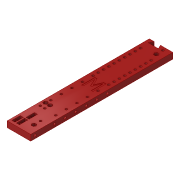
# Autodesk Inventor part: Coupler extension arm motor
Saved by Autodesk Inventor 2020 (Build 240168000, 168)
## iProperties
Created: 2019-10-02
Part Number: Coupler extension arm motor
Material: Generic
Document SubType Name: Modeling
Designer: ball
Density: 1 g/cm^3
Appearance: Default
Author: ball
Autodesk Inventor part; units mm, degrees
ref_plane "YZ Plane" through (0, 0, 0) normal (1, 0, 0) x (0, 1, 0)
ref_plane "XZ Plane" through (0, 0, 0) normal (0, 1, 0) x (-1, 0, 0)
ref_plane "XY Plane" through (0, 0, 0) normal (0, 0, 1) x (1, 0, 0)
sketch "Sketch1" plane through (0, 0, 0) normal (0, 1, 0) x (-1, 0, 0)
  line L0 (0, 0) -> (35.5, 0)
  line L1 (35.5, 0) -> (35.5, -215)
  line L2 (35.5, -215) -> (0, -215)
  line L3 (0, -215) -> (0, 0)
  dimension "d0" = 35.5
  dimension "d1" = 215
  constraints: 8 end point, 2 parallel, 1 horizontal, 1 perpendicular
  measures "d0" distance of L1.end L2.end
  measures "d1" distance of L0.end L1.end
extrude "BlockShape" add sketch "Sketch1" along normal blind 9
sketch "Sketch2" plane through (0, 9, 0) normal (0, 1, 0) x (1, 0, 0)
  circle A0 centre (-10, 15) radius 3.25 construction
  line L0 (-35.5, 0) -> (0, 0) projected
  line L1 (0, 0) -> (0, 215) projected
  line L2 (-13.25, 15) -> (-11.625, 17.8146)
  line L3 (-11.625, 17.8146) -> (-8.375, 17.8146)
  line L4 (-8.375, 17.8146) -> (-6.75, 15)
  line L5 (-6.75, 15) -> (-8.375, 12.1854)
  line L6 (-8.375, 12.1854) -> (-11.625, 12.1854)
  line L7 (-11.625, 12.1854) -> (-13.25, 15)
  circle A1 centre (-10, 200) radius 3.25 construction
  line L8 (-13.25, 200) -> (-11.625, 202.8146)
  line L9 (-11.625, 202.8146) -> (-8.375, 202.8146)
  line L10 (-8.375, 202.8146) -> (-6.75, 200)
  line L11 (-6.75, 200) -> (-8.375, 197.1854)
  line L12 (-8.375, 197.1854) -> (-11.625, 197.1854)
  line L13 (-11.625, 197.1854) -> (-13.25, 200)
  line L14 (0, 215) -> (-35.5, 215) projected
  circle A2 centre (-10, 15) radius 1.7 construction
  circle A3 centre (-10, 200) radius 1.7 construction
  dimension "d7" = 6.5
  dimension "d10" = 6.5
  dimension "d23" = 185
  dimension "d24" = 15
  dimension "d25" = 10
  dimension "d28" = 3.4
  dimension "d29" = 3.4
  constraints: 24 end point, 4 coincident, 2 centre point, 2 horizontal alignment, 30 other
  measures "d23" distance of point (-10, 200) point (-10, 15)
  measures "d24" distance from line of L0 point (-10, 15)
  measures "d25" distance from line of L1 point (-10, 15)
  measures "d28" diameter of A2
  measures "d29" diameter of A3
extrude "SlideNutWell2" cut sketch "Sketch2" against normal blind 5
sketch "Sketch3" plane through (0, 0, 0) normal (0, -1, 0) x (1, 0, 0)
  circle A0 centre (-10, -25) radius 3.25 construction
  line L0 (0, 0) -> (-35.5, 0) projected
  line L1 (-35.5, 0) -> (-35.5, -215) projected
  line L2 (-11.6286, -27.8125) -> (-13.25, -24.9958)
  line L3 (-13.25, -24.9958) -> (-11.6214, -22.1833)
  line L4 (-11.6214, -22.1833) -> (-8.3714, -22.1875)
  line L5 (-8.3714, -22.1875) -> (-6.75, -25.0042)
  line L6 (-6.75, -25.0042) -> (-8.3786, -27.8167)
  line L7 (-8.3786, -27.8167) -> (-11.6286, -27.8125)
  circle A1 centre (-10, -210) radius 3.25 construction
  line L8 (-6.75, -210) -> (-8.375, -212.8146)
  line L9 (-8.375, -212.8146) -> (-11.625, -212.8146)
  line L10 (-11.625, -212.8146) -> (-13.25, -210)
  line L11 (-13.25, -210) -> (-11.625, -207.1854)
  line L12 (-11.625, -207.1854) -> (-8.375, -207.1854)
  line L13 (-8.375, -207.1854) -> (-6.75, -210)
  line L14 (0, -215) -> (0, 0) projected
  dimension "d15" = 6.5
  dimension "d18" = 6.5
  dimension "d16" = 25
  dimension "d19" = 185
  dimension "d26" = 10
  dimension "d27" = 10
  constraints: 24 end point, 2 coincident, 1 horizontal alignment, 31 other
  measures "d16" distance from line of L0 point (-10, -25)
  measures "d19" distance of point (-10, -210) point (-10, -25)
  measures "d26" distance from line of L14 point (-10, -25)
  measures "d27" distance from line of L14 point (-10, -210)
extrude "SlideNutWell1" cut sketch "Sketch3" against normal blind 5
sketch "Sketch5" plane through (0, 9, 0) normal (0, 1, 0) x (1, 0, 0)
  circle A0 centre (-10, 15) radius 1.7
  line L0 (0, 0) -> (0, 215) projected
  line L1 (-35.5, 0) -> (0, 0) projected
  circle A1 centre (-10, 200) radius 1.7
  circle A2 centre (-10, 25) radius 1.7
  circle A3 centre (-10, 210) radius 1.7
  dimension "d30" = 3.4
  dimension "d31" = 10
  dimension "d32" = 15
  dimension "d33" = 3.4
  dimension "d34" = 10
  dimension "d35" = 185
  dimension "d36" = 3.4
  dimension "d37" = 25
  dimension "d38" = 3.4
  dimension "d39" = 10
  dimension "d40" = 185
  constraints: 4 centre point
  measures "d30" diameter of A0
  measures "d31" distance from line of L0 A0.centre
  measures "d32" distance from line of L1 A0.centre
  measures "d33" diameter of A1
  measures "d34" distance from line of L0 A1.centre
  measures "d35" distance of A1.centre A0.centre
  measures "d36" diameter of A2
  measures "d37" distance from line of L1 A2.centre
  measures "d38" diameter of A3
  measures "d39" distance from line of L0 A3.centre
  measures "d40" distance of A2.centre A3.centre
extrude "SlideMoutingHoles" cut sketch "Sketch5" against normal through all
sketch "Sketch6" plane through (0, 9, 0) normal (0, 1, 0) x (1, 0, 0)
  line L0 (-32.5, 4) -> (-27.7502, 4)
  line L1 (-27.7502, 4) -> (-27.7502, 16.7)
  line L2 (-27.7502, 16.7) -> (-32.5, 16.7)
  line L3 (-32.5, 16.7) -> (-32.5, 4)
  line L4 (-35.5, 0) -> (0, 0) projected
  line L5 (-35.5, 215) -> (-35.5, 0) projected
  line L6 (-25.7502, 4) -> (-21.0002, 4)
  line L7 (-21.0002, 4) -> (-21.0002, 16.7)
  line L8 (-21.0002, 16.7) -> (-25.7502, 16.7)
  line L9 (-25.7502, 16.7) -> (-25.7502, 4)
  line L10 (0, 0) -> (0, 215) construction
  line L11 (-35.5, 215) -> (0, 215) projected
  line L12 (0, 0) -> (-20, 0) construction
  line L13 (-20, 0) -> (-20, 215) construction
  line L14 (-20, 215) -> (0, 215) construction
  line L15 (0, 215) -> (0, 0)
  circle A0 centre (-23.3752, 44.7) radius 1.7
  circle A1 centre (-30.125, 44.7) radius 1.7
  circle A2 centre (-30.125, 52.7) radius 1.7
  circle A3 centre (-23.3752, 52.7) radius 1.7
  line L16 (-25.7502, 18.7) -> (-21.0002, 18.7)
  line L17 (-21.0002, 18.7) -> (-21.0002, 31.4)
  line L18 (-21.0002, 31.4) -> (-25.7502, 31.4)
  line L19 (-25.7502, 31.4) -> (-25.7502, 18.7)
  dimension "d43" = 4.7498
  dimension "d44" = 12.7
  dimension "d45" = 4
  dimension "d46" = 3
  dimension "d47" = 4.75
  dimension "d48" = 2
  dimension "d49" = 20
  dimension "d50" = 3.4
  dimension "d51" = 28
  dimension "d87" = 3.4
  dimension "d88" = 5.375
  dimension "d90" = 3.4
  dimension "d91" = 8
  dimension "d92" = 3.4
  dimension "d180" = 4.75
  dimension "d181" = 12.7
  dimension "d182" = 2
  dimension "d183" = 12.7
  dimension "d184" = 4
  dimension "d260" = 28
  dimension "d261" = 8
  constraints: 32 end point, 8 parallel, 4 centre point, 4 horizontal, 4 perpendicular, 2 point on line
  measures "d43" distance of L2.end L1.end
  measures "d44" distance of L1.end L0.end
  measures "d45" distance between parallel lines of L4 L0
  measures "d46" distance between parallel lines of L5 L3
  measures "d47" distance of L8.end L7.end
  measures "d48" distance between parallel lines of L9 L1
  measures "d49" distance of L13.end L14.end
  measures "d50" diameter of A0
  measures "d51" distance from line of A0.centre L8
  measures "d87" diameter of A1
  measures "d88" distance from line of L5 A1.centre
  measures "d90" diameter of A2
  measures "d91" distance of A2.centre A1.centre
  measures "d92" diameter of A3
  measures "d180" distance of L18.end L17.end
  measures "d181" distance of L17.end L16.end
  measures "d182" distance between parallel lines of L16 L8
  measures "d183" distance between parallel lines of L8 L6
  measures "d184" distance between parallel lines of L4 L6
  measures "d260" distance from line of L2 A1.centre
  measures "d261" distance of A0.centre A3.centre
extrude "PulleyHoles" cut sketch "Sketch6" against normal through all contours L3 L2 L1 L0 | L9 L8 L7 L6 | A0 | A1 | A2 | A3 | L19 L18 L17 L16
sketch "Sketch7" plane through (0, 0, 0) normal (0, -1, 0) x (1, 0, 0)
  circle A0 centre (-23.3752, -44.7) radius 1.7 projected
  circle A1 centre (-23.3752, -44.7) radius 3.25 construction
  circle A2 centre (-30.1625, -44.7) radius 3.25 construction
  line L0 (-30.125, -41.4502) -> (-27.3294, -43.1076)
  line L1 (-27.3294, -43.1076) -> (-27.3669, -46.3574)
  line L2 (-27.3669, -46.3574) -> (-30.2, -47.9498)
  line L3 (-30.2, -47.9498) -> (-32.9956, -46.2924)
  line L4 (-32.9956, -46.2924) -> (-32.9581, -43.0426)
  line L5 (-32.9581, -43.0426) -> (-30.125, -41.4502)
  circle A3 centre (-30.125, -44.7) radius 1.7 projected
  line L6 (-20.1252, -44.7) -> (-21.7502, -47.5146)
  line L7 (-21.7502, -47.5146) -> (-25.0002, -47.5146)
  line L8 (-25.0002, -47.5146) -> (-26.6252, -44.7)
  line L9 (-26.6252, -44.7) -> (-25.0002, -41.8854)
  line L10 (-25.0002, -41.8854) -> (-21.7502, -41.8854)
  line L11 (-21.7502, -41.8854) -> (-20.1252, -44.7)
  point P0 (0, 0)
  dimension "d54" = 6.5
  dimension "d89" = 6.5
  dimension "d262" = 0
  constraints: 24 end point, 4 coincident, 1 horizontal alignment, 32 other
  measures "d262" vertical distance of point (-30.162, -44.7) A3.centre
extrude "TensionNutWells2" cut sketch "Sketch7" against normal blind 5 contours A0 | L0 L1 L2 L3 L4 L5 | A3 | L6 L7 L8 L9 L10 L11
sketch "Sketch8" plane through (-35.5, 0, -215) normal (-1, 0, 0) x (0, 0, 1)
  circle A0 centre (204.65, 4.5) radius 1.4605
  line L0 (0, 9) -> (215, 9) projected
  line L1 (215, 0) -> (215, 9) projected
  circle A1 centre (189.95, 4.5) radius 1.45
  dimension "d57" = 2.921
  dimension "d58" = 4.5
  dimension "d59" = 10.35
  dimension "d185" = 2.9
  dimension "d186" = 14.7
  dimension "d187" = 4.5
  constraints: 2 centre point
  measures "d57" diameter of A0
  measures "d58" distance from line of L0 A0.centre
  measures "d59" distance from line of L1 A0.centre
  measures "d185" diameter of A1
  measures "d186" distance of A1.centre A0.centre
  measures "d187" distance from line of L0 A1.centre
hole "PulleyMountingHole" at (-35.5, 4.5, -10.35) at (-35.5, 4.5, -25.05) direction (1, 0, 0) diameter 2.921 depth 21 counterbore diameter 3.4 counterbore depth 1.5
sketch "Sketch9" plane through (-21.0002, 9, -16.7) normal (-1, 0, 0) x (0, 0, 1)
  circle A0 centre (6.35, -4.5) radius 1.4605 projected
  circle A1 centre (6.35, -4.5) radius 2.54
  circle A2 centre (-8.35, -4.5) radius 1.4605 projected
  circle A3 centre (-8.35, -4.5) radius 2.54
  point P0 (16.7, -9)
  dimension "d67" = 5.08
  dimension "d194" = 5.08
  constraints: 2 centre point, 2 coincident
  measures "d67" diameter of A1
  measures "d194" diameter of A3
extrude "PulleyStandoff4" add sketch "Sketch9" along normal blind 0.2032
sketch "Sketch11" plane through (-25.7502, 9, -4) normal (1, 0, 0) x (0, 0, -1)
  circle A0 centre (6.35, -4.5) radius 2.54
  circle A1 centre (6.35, -4.5) radius 1.4605
  circle A2 centre (21.05, -4.5) radius 1.4605 projected
  circle A3 centre (21.05, -4.5) radius 2.54
  point P0 (-4, -9)
  dimension "d73" = 5.08
  dimension "d195" = 5.08
  constraints: 3 centre point, 3 coincident
  measures "d73" diameter of A0
  measures "d195" diameter of A3
sketch "Sketch12" plane through (-32.5, 9, -4) normal (1, 0, 0) x (0, 0, -1)
  circle A0 centre (6.35, -4.5) radius 2.54
  circle A1 centre (6.35, -4.5) radius 1.4605
  point P0 (-4, -9)
  dimension "d76" = 5.08
  constraints: 2 centre point, 1 coincident
  measures "d76" diameter of A0
extrude "PulleyStandoff1" add sketch "Sketch12" along normal blind 0.2032
sketch "Sketch10" plane through (-27.7502, 9, -16.7) normal (-1, 0, 0) x (0, 0, 1)
  circle A0 centre (6.35, -4.5) radius 2.54
  circle A1 centre (6.35, -4.5) radius 1.4605
  point P0 (16.7, -9)
  dimension "d70" = 5.08
  constraints: 2 centre point, 2 coincident
  measures "d70" diameter of A0
extrude "PulleyStandoff2" add sketch "Sketch10" along normal blind 0.2032
extrude "PulleyStandoff3" add sketch "Sketch11" along normal blind 0.2032
sketch "Sketch15" plane through (0, 9, 0) normal (0, 1, 0) x (1, 0, 0)
  circle A0 centre (-30.125, 52.7) radius 1.7 projected
  circle A1 centre (-30.125, 52.7) radius 3.25 construction
  circle A2 centre (-23.3752, 52.7) radius 1.7 projected
  circle A3 centre (-23.3752, 52.7) radius 3.25 construction
  line L0 (-30.125, 49.45) -> (-32.9396, 51.075)
  line L1 (-32.9396, 51.075) -> (-32.9396, 54.325)
  line L2 (-32.9396, 54.325) -> (-30.125, 55.95)
  line L3 (-30.125, 55.95) -> (-27.3104, 54.325)
  line L4 (-27.3104, 54.325) -> (-27.3104, 51.075)
  line L5 (-27.3104, 51.075) -> (-30.125, 49.45)
  line L6 (-23.3752, 49.45) -> (-26.1898, 51.075)
  line L7 (-26.1898, 51.075) -> (-26.1898, 54.325)
  line L8 (-26.1898, 54.325) -> (-23.3752, 55.95)
  line L9 (-23.3752, 55.95) -> (-20.5606, 54.325)
  line L10 (-20.5606, 54.325) -> (-20.5606, 51.075)
  line L11 (-20.5606, 51.075) -> (-23.3752, 49.45)
  point P0 (0, 0)
  dimension "d93" = 6.5
  dimension "d94" = 6.5
  constraints: 24 end point, 4 coincident, 2 vertical alignment, 30 other
extrude "TensionNutWells1" cut sketch "Sketch15" against normal blind 5
ref_plane "PulleyMidPlane1" through (-30.1251, 9, -4) normal (1, 0, 0) x (0, 0, -1)
ref_plane "PulleyMidPlane2" through (-23.3752, 9, -16.7) normal (-1, 0, 0) x (0, 0, 1)
ref_plane "Work Plane3" through (-7.7, 0, 0) normal (1, 0, 0) x (0, 0, -1)
ref_plane "Work Plane4" through (-27.8, 0, -215) normal (-1, 0, 0) x (0, 0, 1)
sketch "Sketch25" plane through (0, 0, 0) normal (0, -1, 0) x (1, 0, 0)
  circle A0 centre (-10, -200) radius 1.75 construction
  circle A1 centre (-10, -25) radius 1.7 construction
  circle A2 centre (-10, -15) radius 1.7 construction
  circle A3 centre (-10, -210) radius 1.7 construction
  line L0 (-35.5, -215) -> (0, -215) construction
  line L1 (0, -215) -> (-35.5, -215) construction
  line L2 (0, -215) -> (-35.5, -215) construction
  line L3 (-23.5, -215) -> (-23.5, -209.55) construction
  line L4 (-18.7502, -215) -> (-15.7022, -208.904)
  line L5 (-15.7022, -208.904) -> (-18.7502, -208.904)
  line L6 (-35.5, -215) -> (0, -215) projected
  line L7 (-28.2498, -215) -> (-31.2978, -208.904)
  line L8 (-27.1, -210.7) -> (-27.1, -207.3) projected
  line L9 (-31.2978, -208.904) -> (-28.2498, -208.904)
  line L10 (-18.7502, -215) -> (-18.7502, -208.904) construction
  line L11 (-28.2498, -215) -> (-28.2498, -208.904) construction
  line L12 (-18.7502, -208.904) -> (-28.2498, -208.904)
  line L13 (-35.5, 0) -> (-35.5, -215) projected
  line L14 (-18.7502, -215) -> (-28.2498, -215)
  point P0 (0, 0)
  point P1 (-15.75, -215)
  point P2 (-20.25, -215)
  dimension "d280" = 10
  dimension "d281" = 3.4
  dimension "d282" = 10
  dimension "d284" = 6.096
  dimension "d285" = 3.048
  dimension "d288" = 3.048
  dimension "d289" = 9.4996
  dimension "d290" = 4.7498
  dimension "d291" = 12
  constraints: 18 end point, 4 horizontal, 3 perpendicular, 2 point on line, 1 centre point, 1 collinear, 2 other
  measures "d280" distance of A1.centre A2.centre
  measures "d281" diameter of A3
  measures "d282" distance of A3.centre A0.centre
  measures "d284" distance between parallel lines of L5 L0
  measures "d285" horizontal distance of L4.end L4.start
  measures "d288" horizontal distance of L7.end L7.start
  measures "d289" distance of L7.start L4.start
  measures "d290" distance from line of L7.start L3
  measures "d291" distance between parallel lines of L13 L3
extrude "Extrusion22" cut sketch "Sketch25" against normal through all
sketch "Sketch26" plane through (0, 9, 0) normal (0, 1, 0) x (1, 0, 0)
  circle A0 centre (-29.75, 204) radius 1.7 construction
  circle A1 centre (-29.75, 220) radius 1.7 construction
  circle A2 centre (-5.75, 220) radius 1.7 construction
  line L0 (-35.5, 215) -> (-35.5, 0) construction
  circle A3 centre (-29.75, 196) radius 1.7
  circle A4 centre (-29.75, 188) radius 1.7
  circle A5 centre (-5.75, 188) radius 1.7
  line L1 (0, 0) -> (0, 215) projected
  circle A6 centre (-29.75, 180) radius 1.7
  circle A7 centre (-5.75, 180) radius 1.7
  circle A8 centre (-29.75, 172) radius 1.7
  circle A9 centre (-5.75, 172) radius 1.7
  circle A10 centre (-29.75, 164) radius 1.7
  circle A11 centre (-5.75, 164) radius 1.7
  circle A12 centre (-29.75, 156) radius 1.7
  circle A13 centre (-5.75, 156) radius 1.7
  circle A14 centre (-29.75, 148) radius 1.7
  circle A15 centre (-5.75, 148) radius 1.7
  circle A16 centre (-29.75, 140) radius 1.7
  circle A17 centre (-5.75, 140) radius 1.7
  circle A18 centre (-29.75, 132) radius 1.7
  circle A19 centre (-5.75, 132) radius 1.7
  dimension "d294" = 3.4
  dimension "d295" = 16
  dimension "d296" = 5.75
  dimension "d297" = 3.4
  dimension "d298" = 8
  dimension "d299" = 3.4
  dimension "d300" = 8
  dimension "d301" = 5.75
  dimension "d302" = 3.4
  dimension "d303" = 5.75
  dimension "d304" = 32
  dimension "d307" = 8
  constraints: 20 centre point, 1 vertical, 32 other
  measures "d294" diameter of A0
  measures "d295" distance of A0.centre A1.centre
  measures "d296" distance from line of L0 A0.centre
  measures "d297" diameter of A3
  measures "d298" distance of A0.centre A3.centre
  measures "d299" diameter of A4
  measures "d300" distance of A3.centre A4.centre
  measures "d301" distance from line of L0 A4.centre
  measures "d302" diameter of A5
  measures "d303" distance from line of L1 A5.centre
  measures "d304" distance of A2.centre A5.centre
  measures "d307" distance of A4.centre A6.centre
extrude "CrossBarMoutingHoles" cut sketch "Sketch26" against normal through all
sketch "Sketch27" plane through (0, 0, 0) normal (0, -1, 0) x (1, 0, 0)
  circle A0 centre (-5.75, -188) radius 1.7 construction
  circle A1 centre (-5.75, -188) radius 3.25 construction
  circle A2 centre (-29.75, -196) radius 1.7 construction
  circle A3 centre (-29.75, -196) radius 3.25 construction
  circle A4 centre (-29.75, -188) radius 1.7 construction
  circle A5 centre (-29.75, -188) radius 3.25 construction
  line L0 (-9, -188) -> (-7.375, -185.1854)
  line L1 (-7.375, -185.1854) -> (-4.125, -185.1854)
  line L2 (-4.125, -185.1854) -> (-2.5, -188)
  line L3 (-2.5, -188) -> (-4.125, -190.8146)
  line L4 (-4.125, -190.8146) -> (-7.375, -190.8146)
  line L5 (-7.375, -190.8146) -> (-9, -188)
  line L6 (-33, -188) -> (-31.375, -185.1854)
  line L7 (-31.375, -185.1854) -> (-28.125, -185.1854)
  line L8 (-28.125, -185.1854) -> (-26.5, -188)
  line L9 (-26.5, -188) -> (-28.125, -190.8146)
  line L10 (-28.125, -190.8146) -> (-31.375, -190.8146)
  line L11 (-31.375, -190.8146) -> (-33, -188)
  line L12 (-26.5, -196) -> (-28.125, -198.8146)
  line L13 (-28.125, -198.8146) -> (-31.375, -198.8146)
  line L14 (-31.375, -198.8146) -> (-33, -196)
  line L15 (-33, -196) -> (-31.375, -193.1854)
  line L16 (-31.375, -193.1854) -> (-28.125, -193.1854)
  line L17 (-28.125, -193.1854) -> (-26.5, -196)
  line L18 (0, -215) -> (0, 0) construction
  line L19 (-26.5, -180) -> (-28.125, -182.8146)
  line L20 (-31.375, -182.8146) -> (-33, -180)
  circle A6 centre (-29.75, -180) radius 3.25 construction
  line L21 (-28.125, -177.1854) -> (-26.5, -180)
  line L22 (-31.375, -177.1854) -> (-28.125, -177.1854)
  line L23 (-33, -180) -> (-31.375, -177.1854)
  circle A7 centre (-5.75, -180) radius 3.25 construction
  line L24 (-9, -180) -> (-7.375, -177.1854)
  line L25 (-7.375, -182.8146) -> (-9, -180)
  line L26 (-7.375, -177.1854) -> (-4.125, -177.1854)
  line L27 (-2.5, -180) -> (-4.125, -182.8146)
  line L28 (-4.125, -177.1854) -> (-2.5, -180)
  line L29 (-4.125, -182.8146) -> (-7.375, -182.8146)
  line L30 (-28.125, -182.8146) -> (-31.375, -182.8146)
  line L31 (-26.5, -172) -> (-28.125, -174.8146)
  line L32 (-31.375, -174.8146) -> (-33, -172)
  circle A8 centre (-29.75, -172) radius 3.25 construction
  line L33 (-28.125, -169.1854) -> (-26.5, -172)
  line L34 (-31.375, -169.1854) -> (-28.125, -169.1854)
  line L35 (-33, -172) -> (-31.375, -169.1854)
  circle A9 centre (-5.75, -172) radius 3.25 construction
  line L36 (-9, -172) -> (-7.375, -169.1854)
  line L37 (-7.375, -174.8146) -> (-9, -172)
  line L38 (-7.375, -169.1854) -> (-4.125, -169.1854)
  line L39 (-2.5, -172) -> (-4.125, -174.8146)
  line L40 (-4.125, -169.1854) -> (-2.5, -172)
  line L41 (-4.125, -174.8146) -> (-7.375, -174.8146)
  line L42 (-28.125, -174.8146) -> (-31.375, -174.8146)
  line L43 (-26.5, -164) -> (-28.125, -166.8146)
  line L44 (-31.375, -166.8146) -> (-33, -164)
  circle A10 centre (-29.75, -164) radius 3.25 construction
  line L45 (-28.125, -161.1854) -> (-26.5, -164)
  line L46 (-31.375, -161.1854) -> (-28.125, -161.1854)
  line L47 (-33, -164) -> (-31.375, -161.1854)
  circle A11 centre (-5.75, -164) radius 3.25 construction
  line L48 (-9, -164) -> (-7.375, -161.1854)
  line L49 (-7.375, -166.8146) -> (-9, -164)
  line L50 (-7.375, -161.1854) -> (-4.125, -161.1854)
  line L51 (-2.5, -164) -> (-4.125, -166.8146)
  line L52 (-4.125, -161.1854) -> (-2.5, -164)
  line L53 (-4.125, -166.8146) -> (-7.375, -166.8146)
  line L54 (-28.125, -166.8146) -> (-31.375, -166.8146)
  line L55 (-26.5, -156) -> (-28.125, -158.8146)
  line L56 (-31.375, -158.8146) -> (-33, -156)
  circle A12 centre (-29.75, -156) radius 3.25 construction
  line L57 (-28.125, -153.1854) -> (-26.5, -156)
  line L58 (-31.375, -153.1854) -> (-28.125, -153.1854)
  line L59 (-33, -156) -> (-31.375, -153.1854)
  circle A13 centre (-5.75, -156) radius 3.25 construction
  line L60 (-9, -156) -> (-7.375, -153.1854)
  line L61 (-7.375, -158.8146) -> (-9, -156)
  line L62 (-7.375, -153.1854) -> (-4.125, -153.1854)
  line L63 (-2.5, -156) -> (-4.125, -158.8146)
  line L64 (-4.125, -153.1854) -> (-2.5, -156)
  line L65 (-4.125, -158.8146) -> (-7.375, -158.8146)
  line L66 (-28.125, -158.8146) -> (-31.375, -158.8146)
  line L67 (-26.5, -148) -> (-28.125, -150.8146)
  line L68 (-31.375, -150.8146) -> (-33, -148)
  circle A14 centre (-29.75, -148) radius 3.25 construction
  line L69 (-28.125, -145.1854) -> (-26.5, -148)
  line L70 (-31.375, -145.1854) -> (-28.125, -145.1854)
  line L71 (-33, -148) -> (-31.375, -145.1854)
  circle A15 centre (-5.75, -148) radius 3.25 construction
  line L72 (-9, -148) -> (-7.375, -145.1854)
  line L73 (-7.375, -150.8146) -> (-9, -148)
  line L74 (-7.375, -145.1854) -> (-4.125, -145.1854)
  line L75 (-2.5, -148) -> (-4.125, -150.8146)
  line L76 (-4.125, -145.1854) -> (-2.5, -148)
  line L77 (-4.125, -150.8146) -> (-7.375, -150.8146)
  line L78 (-28.125, -150.8146) -> (-31.375, -150.8146)
  line L79 (-26.5, -140) -> (-28.125, -142.8146)
  line L80 (-31.375, -142.8146) -> (-33, -140)
  circle A16 centre (-29.75, -140) radius 3.25 construction
  line L81 (-28.125, -137.1854) -> (-26.5, -140)
  line L82 (-31.375, -137.1854) -> (-28.125, -137.1854)
  line L83 (-33, -140) -> (-31.375, -137.1854)
  circle A17 centre (-5.75, -140) radius 3.25 construction
  line L84 (-9, -140) -> (-7.375, -137.1854)
  line L85 (-7.375, -142.8146) -> (-9, -140)
  line L86 (-7.375, -137.1854) -> (-4.125, -137.1854)
  line L87 (-2.5, -140) -> (-4.125, -142.8146)
  line L88 (-4.125, -137.1854) -> (-2.5, -140)
  line L89 (-4.125, -142.8146) -> (-7.375, -142.8146)
  line L90 (-28.125, -142.8146) -> (-31.375, -142.8146)
  line L91 (-26.5, -132) -> (-28.125, -134.8146)
  line L92 (-31.375, -134.8146) -> (-33, -132)
  circle A18 centre (-29.75, -132) radius 3.25 construction
  line L93 (-28.125, -129.1854) -> (-26.5, -132)
  line L94 (-31.375, -129.1854) -> (-28.125, -129.1854)
  line L95 (-33, -132) -> (-31.375, -129.1854)
  circle A19 centre (-5.75, -132) radius 3.25 construction
  line L96 (-9, -132) -> (-7.375, -129.1854)
  line L97 (-7.375, -134.8146) -> (-9, -132)
  line L98 (-7.375, -129.1854) -> (-4.125, -129.1854)
  line L99 (-2.5, -132) -> (-4.125, -134.8146)
  line L100 (-4.125, -129.1854) -> (-2.5, -132)
  line L101 (-4.125, -134.8146) -> (-7.375, -134.8146)
  line L102 (-28.125, -134.8146) -> (-31.375, -134.8146)
  dimension "d314" = 6.5
  dimension "d315" = 6.5
  dimension "d316" = 6.5
  dimension "d319" = 8
  constraints: 204 end point, 34 coincident, 17 horizontal alignment, 15 vertical, 283 other
  measures "d319" distance of L9.end L19.end
extrude "CrossBarNutWells" cut sketch "Sketch27" against normal blind 5
ref_plane "Work Plane5" through (-19, 0, -215) normal (-1, 0, 0) x (0, 0, 1)
sketch "Sketch28" plane through (-19, 0, -215) normal (-1, 0, 0) x (0, 0, 1)
  circle A0 centre (204.65, 4.5) radius 1.4605 construction
  circle A1 centre (204.65, 4.5) radius 3.45 construction
  line L0 (204.65, 7.95) -> (207.6378, 6.225)
  line L1 (207.6378, 6.225) -> (207.6378, 0)
  line L2 (201.6622, 0) -> (201.6622, 6.225)
  line L3 (201.6622, 6.225) -> (204.65, 7.95)
  line L4 (0, 0) -> (215, 0) projected
  line L5 (207.6378, 0) -> (201.6622, 0)
  circle A2 centre (189.95, 4.5) radius 1.4605 projected
  circle A3 centre (189.95, 4.5) radius 3.45 construction
  line L6 (189.95, 7.95) -> (192.9378, 6.225)
  line L7 (192.9378, 6.225) -> (192.9378, 0)
  line L8 (186.9622, 0) -> (186.9622, 6.225)
  line L9 (186.9622, 6.225) -> (189.95, 7.95)
  line L10 (192.9378, 0) -> (186.9622, 0)
  dimension "d327" = 6.9
  dimension "d328" = 6.9
  constraints: 20 end point, 3 coincident, 2 point on line, 2 vertical alignment, 16 other
extrude "PullyNetWells" cut sketch "Sketch28" against normal blind 2.8
sketch "Sketch29" plane through (0, 0, 0) normal (1, 0, 0) x (0, 0, -1)
  line L0 (0, 9) -> (215, 9) projected
  line L1 (215, 0) -> (0, 0) projected
  circle A0 centre (6.5, 4.5) radius 1.7
  line L2 (13.3, 4) -> (13.3, 0) construction
  line L3 (0, 0) -> (0, 9) construction
  line L4 (28.0378, 0) -> (28.0378, 6.225) construction
  line L5 (129.1854, 0) -> (129.1854, 5) construction
  circle A1 centre (36, 4.5) radius 1.7
  circle A2 centre (52, 4.5) radius 1.7
  circle A3 centre (68, 4.5) radius 1.7
  circle A4 centre (84, 4.5) radius 1.7
  circle A5 centre (100, 4.5) radius 1.7
  circle A6 centre (116, 4.5) radius 1.7
  dimension "d331" = 9
  dimension "d332" = 3.4
  dimension "d333" = 4.5
  dimension "d334" = 6.5
  dimension "d335" = 3.4
  dimension "d336" = 4.5
  dimension "d337" = 36
  dimension "d340" = 16
  constraints: 7 centre point, 1 horizontal, 10 other
  measures "d331" distance between parallel lines of L0 L1
  measures "d332" diameter of A0
  measures "d333" distance from line of L0 A0.centre
  measures "d334" distance from line of L3 A0.centre
  measures "d335" diameter of A1
  measures "d336" distance from line of L0 A1.centre
  measures "d337" distance from line of L3 A1.centre
  measures "d340" distance of A1.centre A2.centre
extrude "SideHolesNonPulley" cut sketch "Sketch29" against normal blind 8.4
ref_plane "Work Plane6" through (-7.7, 0, 0) normal (1, 0, 0) x (0, 0, -1)
sketch "Sketch30" plane through (-7.7, 0, 0) normal (1, 0, 0) x (0, 0, -1)
  circle A0 centre (36, 4.5) radius 1.7 construction
  circle A1 centre (36, 4.5) radius 3.45 construction
  line L0 (36, 7.95) -> (38.9878, 6.225)
  line L1 (38.9878, 6.225) -> (38.9878, 0)
  line L2 (33.0122, 0) -> (33.0122, 6.225)
  line L3 (33.0122, 6.225) -> (36, 7.95)
  line L4 (0, 0) -> (215, 0) projected
  line L5 (38.9878, 0) -> (33.0122, 0)
  circle A2 centre (6.5, 4.5) radius 3.45 construction
  line L6 (6.5, 7.95) -> (9.4878, 6.225)
  line L7 (9.4878, 6.225) -> (9.4878, 0)
  line L8 (3.5122, 0) -> (3.5122, 6.225)
  line L9 (3.5122, 6.225) -> (6.5, 7.95)
  line L10 (9.4878, 0) -> (3.5122, 0)
  line L11 (49.0122, 0) -> (49.0122, 6.225)
  line L12 (49.0122, 6.225) -> (52, 7.95)
  line L13 (54.9878, 6.225) -> (54.9878, 0)
  line L14 (54.9878, 0) -> (49.0122, 0)
  circle A3 centre (52, 4.5) radius 3.45 construction
  line L15 (52, 7.95) -> (54.9878, 6.225)
  line L16 (65.0122, 0) -> (65.0122, 6.225)
  line L17 (65.0122, 6.225) -> (68, 7.95)
  line L18 (70.9878, 6.225) -> (70.9878, 0)
  line L19 (70.9878, 0) -> (65.0122, 0)
  circle A4 centre (68, 4.5) radius 3.45 construction
  line L20 (68, 7.95) -> (70.9878, 6.225)
  line L21 (81.0122, 0) -> (81.0122, 6.225)
  line L22 (81.0122, 6.225) -> (84, 7.95)
  line L23 (86.9878, 6.225) -> (86.9878, 0)
  line L24 (86.9878, 0) -> (81.0122, 0)
  circle A5 centre (84, 4.5) radius 3.45 construction
  line L25 (84, 7.95) -> (86.9878, 6.225)
  line L26 (97.0122, 0) -> (97.0122, 6.225)
  line L27 (97.0122, 6.225) -> (100, 7.95)
  line L28 (102.9878, 6.225) -> (102.9878, 0)
  line L29 (102.9878, 0) -> (97.0122, 0)
  circle A6 centre (100, 4.5) radius 3.45 construction
  line L30 (100, 7.95) -> (102.9878, 6.225)
  line L31 (113.0122, 0) -> (113.0122, 6.225)
  line L32 (113.0122, 6.225) -> (116, 7.95)
  line L33 (118.9878, 6.225) -> (118.9878, 0)
  line L34 (118.9878, 0) -> (113.0122, 0)
  circle A7 centre (116, 4.5) radius 3.45 construction
  line L35 (116, 7.95) -> (118.9878, 6.225)
  point P0 (6.5, 4.5)
  dimension "d349" = 6.9
  dimension "d350" = 6.9
  dimension "d353" = 16
  constraints: 70 end point, 12 coincident, 7 vertical alignment, 6 horizontal, 2 point on line, 91 other
  measures "d353" distance of L2.end L11.end
extrude "SideNutWellsNonPulley" cut sketch "Sketch30" along normal blind 4.4
sketch "Sketch31" plane through (-35.5, 0, -215) normal (-1, 0, 0) x (0, 0, 1)
  circle A0 centre (179, 4.5) radius 1.7
  line L0 (215, 0) -> (215, 9) projected
  line L1 (0, 9) -> (215, 9) projected
  line L2 (215, 0) -> (0, 0) projected
  circle A1 centre (163, 4.5) radius 1.7
  circle A2 centre (147, 4.5) radius 1.7
  circle A3 centre (131, 4.5) radius 1.7
  circle A4 centre (115, 4.5) radius 1.7
  circle A5 centre (99, 4.5) radius 1.7
  dimension "d360" = 3.4
  dimension "d361" = 36
  dimension "d362" = 9
  dimension "d363" = 4.5
  dimension "d366" = 16
  constraints: 6 centre point, 1 horizontal, 10 other
  measures "d360" diameter of A0
  measures "d361" distance from line of L0 A0.centre
  measures "d362" distance between parallel lines of L1 L2
  measures "d363" distance from line of L1 A0.centre
  measures "d366" distance of A0.centre A1.centre
extrude "SideHolesPulleySide" cut sketch "Sketch31" against normal blind 8.4 contours A0 | A2 | A3 | A4 | A5
ref_plane "Work Plane7" through (-27.8, 0, -215) normal (-1, 0, 0) x (0, 0, 1)
sketch "Sketch32" plane through (-27.8, 0, -215) normal (-1, 0, 0) x (0, 0, 1)
  circle A0 centre (147, 4.5) radius 1.7 construction
  circle A1 centre (147, 4.5) radius 3.45 construction
  line L0 (147, 7.95) -> (149.9878, 6.225) projected
  line L1 (147, 7.95) -> (149.9878, 6.225)
  line L2 (149.9878, 6.225) -> (149.9878, 0)
  line L3 (144.0122, 0) -> (144.0122, 6.225)
  line L4 (144.0122, 6.225) -> (147, 7.95)
  line L5 (149.9878, 6.225) -> (149.9878, 0) projected
  line L6 (149.9878, 0) -> (144.0122, 0)
  line L7 (0, 0) -> (215, 0) projected
  circle A2 centre (131, 4.5) radius 3.45 construction
  line L8 (131, 7.95) -> (133.9878, 6.225)
  line L9 (133.9878, 6.225) -> (133.9878, 0)
  line L10 (128.0122, 0) -> (128.0122, 6.225)
  line L11 (128.0122, 6.225) -> (131, 7.95)
  line L12 (133.9878, 0) -> (128.0122, 0)
  circle A3 centre (115, 4.5) radius 3.45 construction
  line L13 (115, 7.95) -> (117.9878, 6.225)
  line L14 (117.9878, 6.225) -> (117.9878, 0)
  line L15 (112.0122, 0) -> (112.0122, 6.225)
  line L16 (112.0122, 6.225) -> (115, 7.95)
  line L17 (117.9878, 0) -> (112.0122, 0)
  circle A4 centre (99, 4.5) radius 3.45 construction
  line L18 (99, 7.95) -> (101.9878, 6.225)
  line L19 (101.9878, 6.225) -> (101.9878, 0)
  line L20 (96.0122, 0) -> (96.0122, 6.225)
  line L21 (96.0122, 6.225) -> (99, 7.95)
  line L22 (101.9878, 0) -> (96.0122, 0)
  circle A5 centre (179, 4.5) radius 1.7 construction
  circle A6 centre (179, 4.5) radius 3.45 construction
  circle A7 centre (179, 4.5) radius 3.45 construction
  line L23 (179, 7.95) -> (181.9878, 6.225)
  line L24 (181.9878, 6.225) -> (181.9878, 0)
  line L25 (176.0122, 0) -> (176.0122, 6.225)
  line L26 (176.0122, 6.225) -> (179, 7.95)
  line L27 (181.9878, 0) -> (176.0122, 0)
  point P0 (133.9878, 6.225)
  point P1 (117.9878, 6.225)
  point P2 (101.9878, 6.225)
  dimension "d387" = 6.9
  dimension "d374" = 6.9
  dimension "d377" = 16
  dimension "d382" = 6.9
  constraints: 50 end point, 9 coincident, 5 centre point, 2 point on line, 1 horizontal, 1 vertical alignment, 61 other
  measures "d374" diameter of A1
  measures "d377" distance of A1.centre A2.centre
  measures "d382" diameter of A6
extrude "SideNutWellsPulleySide" cut sketch "Sketch32" along normal blind 4.4
sketch "Sketch33" plane through (0, 0, 0) normal (0, -1, 0) x (1, 0, 0)
  circle A0 centre (-6, -44) radius 1.7
  line L0 (0, -215) -> (0, 0) projected
  line L1 (0, 0) -> (-35.5, 0) projected
  circle A1 centre (-6, -60) radius 1.7
  circle A2 centre (-29.5, -60) radius 1.7
  line L2 (-35.5, 0) -> (-35.5, -215) projected
  circle A3 centre (-6, -76) radius 1.7
  circle A4 centre (-29.5, -76) radius 1.7
  circle A5 centre (-6, -92) radius 1.7
  circle A6 centre (-29.5, -92) radius 1.7
  circle A7 centre (-6, -108) radius 1.7
  circle A8 centre (-29.5, -108) radius 1.7
  circle A9 centre (-6, -124) radius 1.7
  circle A10 centre (-29.5, -124) radius 1.7
  dimension "d390" = 3.4
  dimension "d391" = 6
  dimension "d392" = 44
  dimension "d393" = 3.4
  dimension "d394" = 16
  dimension "d395" = 6
  dimension "d396" = 3.4
  dimension "d397" = 6
  dimension "d398" = 60
  dimension "d401" = 16
  constraints: 11 centre point, 1 vertical, 16 other
  measures "d390" diameter of A0
  measures "d391" distance from line of L0 A0.centre
  measures "d392" distance from line of L1 A0.centre
  measures "d393" diameter of A1
  measures "d394" distance of A1.centre A0.centre
  measures "d395" distance from line of L0 A1.centre
  measures "d396" diameter of A2
  measures "d397" distance from line of L2 A2.centre
  measures "d398" distance from line of L1 A2.centre
  measures "d401" distance of A1.centre A3.centre
extrude "TieWrapHoles" cut sketch "Sketch33" against normal through all
sketch "Sketch34" plane through (0, 0, 0) normal (0, -1, 0) x (1, 0, 0)
  line L0 (-25.5124, -67.1702) -> (-10.4761, -67.1702) construction
  line L1 (-10.4761, -67.1702) -> (-10.4761, -88.9851) construction
  line L2 (-10.4761, -88.9851) -> (-25.5124, -88.9851) construction
  line L3 (-25.5124, -88.9851) -> (-25.5124, -67.1702) construction
  line L4 (-9.4205, -88.0777) -> (-12.0785, -88.0777)
  line L5 (-12.0785, -88.0777) -> (-12.0785, -70.8492)
  line L6 (-12.0785, -70.8492) -> (-17.2973, -82.5672)
  line L7 (-17.2973, -82.5672) -> (-18.9181, -82.5672)
  line L8 (-18.9181, -82.5672) -> (-24.0882, -70.8492)
  line L9 (-24.0882, -70.8492) -> (-24.0882, -88.0777)
  line L10 (-24.0882, -88.0777) -> (-26.568, -88.0777)
  line L11 (-26.568, -88.0777) -> (-26.568, -68.0777)
  line L12 (-26.568, -68.0777) -> (-22.9375, -68.0777)
  line L13 (-22.9375, -68.0777) -> (-17.9456, -79.2122)
  line L14 (-17.9456, -79.2122) -> (-13.1158, -68.0777)
  line L15 (-13.1158, -68.0777) -> (-9.4205, -68.0777)
  line L16 (-9.4205, -68.0777) -> (-9.4205, -88.0777)
  point P0 (0, 0)
  constraints: 2 other
emboss "Emboss1" sketch "Sketch34" operation cut depth 0.5 direction (0, 1, 0)
sketch "Sketch35" plane through (0, 9, 0) normal (0, 1, 0) x (1, 0, 0)
  line L0 (-25.3891, 123.8644) -> (-9.7366, 123.8644) construction
  line L1 (-9.7366, 123.8644) -> (-9.7366, 102.6657) construction
  line L2 (-9.7366, 102.6657) -> (-25.3891, 102.6657) construction
  line L3 (-25.3891, 102.6657) -> (-25.3891, 123.8644) construction
  line L4 (-8.9891, 103.265) -> (-11.6471, 103.265)
  line L5 (-11.6471, 103.265) -> (-11.6471, 120.4936)
  line L6 (-11.6471, 120.4936) -> (-16.8659, 108.7756)
  line L7 (-16.8659, 108.7756) -> (-18.4867, 108.7756)
  line L8 (-18.4867, 108.7756) -> (-23.6569, 120.4936)
  line L9 (-23.6569, 120.4936) -> (-23.6569, 103.265)
  line L10 (-23.6569, 103.265) -> (-26.1366, 103.265)
  line L11 (-26.1366, 103.265) -> (-26.1366, 123.265)
  line L12 (-26.1366, 123.265) -> (-22.5061, 123.265)
  line L13 (-22.5061, 123.265) -> (-17.5142, 112.1305)
  line L14 (-17.5142, 112.1305) -> (-12.6844, 123.265)
  line L15 (-12.6844, 123.265) -> (-8.9891, 123.265)
  line L16 (-8.9891, 123.265) -> (-8.9891, 103.265)
  point P0 (0, 0)
  constraints: 2 other
emboss "Emboss2" sketch "Sketch35" operation cut depth 0.5 direction (0, -1, 0)
equation "\"d183\" = d44"
equation "\"d184\" = d45"
equation "\"d260\" = d51"
equation "\"d261\" = d91"
equation "\"d187\" = d58"
equation "\"d282\" = d280"
body "Solid1"
